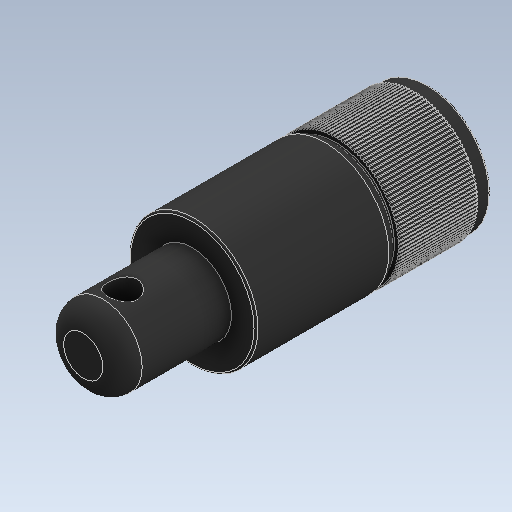
# Autodesk Inventor part: LAIRD_001-0012
Saved by Autodesk Inventor 2021 (Build 250183000, 183)
## iProperties
Created: 2020-06-10
Part Number: LAIRD_001-0012
Material: Generic
Document SubType Name: Modeling
Designer: lgnds
Density: 1 g/cm^3
Appearance: Default
Author: lgnds
Autodesk Inventor part; units mm, degrees
ref_plane "YZ Plane" through (0, 0, 0) normal (1, 0, 0) x (0, 1, 0)
ref_plane "XZ Plane" through (0, 0, 0) normal (0, 1, 0) x (-1, 0, 0)
sketch "Sketch1" plane through (0, 0, 0) normal (0, 0, 1) x (1, 0, 0)
  circle A0 centre (0, 0) radius 6.5
  dimension "d0" = 13
  constraints: 1 centre point, 1 coincident
  measures "d0" diameter of A0
extrude "Extrusion1" add sketch "Sketch1" along normal blind 24.1
sketch "Sketch2" plane through (0, 0, 0) normal (0, 0, -1) x (-1, 0, 0)
  circle A0 centre (0, 0) radius 6.35
  circle A1 centre (0, 0) radius 6.5 projected
  dimension "d3" = 12.7
  constraints: 1 centre point, 1 coincident
  measures "d3" diameter of A0
extrude "Extrusion2" cut sketch "Sketch2" against normal blind 1.5
ref_plane "Work Plane1" through (0, 0, 9.5) normal (0, 0, -1) x (-1, 0, 0)
sketch "Sketch4" plane through (0, 0, 9.5) normal (0, 0, -1) x (-1, 0, 0)
  circle A0 centre (0, 0) radius 6
  circle A1 centre (0, 0) radius 6.5 projected
  dimension "d7" = 0.5
  constraints: 1 centre point, 1 coincident
  measures "d7" radial gap between concentric circles of A1 A0
extrude "Extrusion3" cut sketch "Sketch4" against normal blind 0.2
fillet "Fillet1" radius 1 1 edges at (-6.5, 0, 9.7)
sketch "Sketch5" plane through (0, 0, 1.5) normal (0, 0, -1) x (-1, 0, 0)
  circle A0 centre (0, 0) radius 6.5 projected
  circle A1 centre (6.5, 0) radius 0.125
  dimension "d11" = 0.25
  constraints: 1 centre point, 1 horizontal alignment, 1 other
  measures "d11" diameter of A1
extrude "Extrusion4" cut sketch "Sketch5" against normal up to surface (8 mm away) contours A0 A1 | A0 A1 picked at (6.4198, -0.0159) picked at (6.5801, -0.016)
pattern_circular "Circular Pattern1" count 120 over 360 about axis through (0, 0, 0) along (0, 0, 1) of "Extrusion4"
sketch "Sketch6" plane through (0, 0, 24.1) normal (0, 0, 1) x (1, 0, 0)
  circle A0 centre (0, 0) radius 4
  dimension "d18" = 8
  constraints: 1 centre point, 1 coincident
  measures "d18" diameter of A0
extrude "Extrusion5" add sketch "Sketch6" along normal blind 11.1
sketch "Sketch7" plane through (0, 0, 0) normal (0, 1, 0) x (-1, 0, 0)
  line L0 (0, -7.04) -> (0, 42.24) projected
  circle A0 centre (0, 31.2) radius 1.5
  line L1 (-6.35, 0) -> (6.35, 0) projected
  point P0 (0, 0)
  dimension "d21" = 3
  dimension "d22" = 31.2
  constraints: 1 centre point, 1 point on line
  measures "d21" diameter of A0
  measures "d22" distance from line of L1 A0.centre
extrude "Extrusion6" cut sketch "Sketch7" along normal through all both and the other way through all
fillet "Fillet2" radius 2 1 edges at (-4, 0, 35.2)
fillet "Fillet3" radius 0.2 2 edges at (6.35, 0, 0) (-6.5, 0, 24.1)
body "Solid1"
